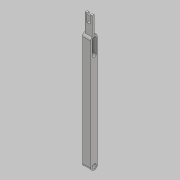
# Autodesk Inventor part: 支架4-15
Saved by Autodesk Inventor 2018 (Build 220112000, 112)
## iProperties
Created: 2021-03-05
Part Number: 支架4-15
Material: 一般
Document SubType Name: Modeling
Designer: 王鼎鈞
Density: 1 g/cm^3
Appearance: 預設
Mass: 2.43299 g
Surface Area: 19.7834 cm^2
Volume: 2.43299 cm^3
Author: 王鼎鈞
Autodesk Inventor part; units mm, degrees
ref_plane "YZ Plane" through (0, 0, 0) normal (1, 0, 0) x (0, 1, 0)
ref_plane "XZ Plane" through (0, 0, 0) normal (0, 1, 0) x (-1, 0, 0)
ref_plane "XY Plane" through (0, 0, 0) normal (0, 0, 1) x (1, 0, 0)
sketch "草圖1" plane through (0, 0, 0) normal (1, 0, 0) x (0, 1, 0)
  line L0 (0, 0) -> (5, 0)
  line L1 (5, 0) -> (5, -85)
  line L2 (5, -85) -> (0, -85)
  line L3 (0, -85) -> (0, 0)
  dimension "d0" = 5
  dimension "d1" = 85
  constraints: 8 end point, 2 parallel, 1 horizontal, 1 perpendicular
  measures "d0" distance of L1.end L2.end
  measures "d1" distance of L0.end L1.end
extrude "擠出1" add sketch "草圖1" along normal blind 6
fillet "圓角1" radius 2.5 2 edges at (3, 5, 0) (3, 0, 0)
hole "孔1" at (6, 2.5, -2.5) direction (-1, 0, 0) diameter 3 end through all
fillet "圓角2" radius 2.5 2 edges at (3, 5, -85) (3, 0, -85)
hole "孔2" at (6, 2.5, -82.5) direction (-1, 0, 0) diameter 3 end through all
sketch "草圖2" plane through (6, 0, 0) normal (1, 0, 0) x (0, 0, -1)
  line L0 (0, -1) -> (0, 6) projected
  line L1 (0, -1) -> (0, 6) projected
  line L2 (120, 0) -> (-20, 0) projected
  circle A0 centre (82.5, 2.5) radius 1.5 projected
  circle A1 centre (2.5, 2.5) radius 1.5 projected
  arc A2 (82.5, 0) -> (82.5, 5) centre (82.5, 2.5) ccw projected
  line L3 (82.5, 5) -> (2.5, 5) projected
  arc A3 (2.5, 5) -> (2.5, 0) centre (2.5, 2.5) ccw projected
  line L4 (2.5, 0) -> (82.5, 0) projected
  circle A4 centre (98.5, 2.5) radius 1.5
  circle A5 centre (82.5, 2.5) radius 1.5 projected
  line L5 (84.5, 4) -> (98.5, 4)
  line L6 (98.5, 4) -> (98.5, 1)
  line L7 (98.5, 1) -> (84.5, 1)
  point P0 (0, 0)
  dimension "d24" = 3
  dimension "d25" = 16
  constraints: 6 end point, 2 point on circle, 1 horizontal, 1 parallel, 1 perpendicular, 1 vertical alignment, 2 other
  measures "d25" distance of A0.centre point (98.5, 2.5)
extrude "擠出2" add sketch "草圖2" against normal blind 5 contours A2 L5 A4 L7 | L6 A4 | A4 L6
ref_plane "工作平面1" through (3, 0, 0) normal (1, 0, 0) x (0, 0, -1)
sketch "草圖3" plane through (3, 0, 0) normal (1, 0, 0) x (0, 0, -1)
  arc A0 (98.5, 1) -> (98.5, 4) centre (98.5, 2.5) ccw projected
  line L0 (98.5, 1) -> (102.8586, 1)
  line L1 (102.8586, 1) -> (102.8586, 5.3685)
  line L2 (102.8586, 5.3685) -> (98.5, 5.3685)
  line L3 (98.5, 5.3685) -> (98.5, 1)
  point P0 (0, 0)
  constraints: 8 end point, 2 parallel, 1 perpendicular
extrude "擠出3" cut sketch "草圖3" along normal mid plane 6
sketch "草圖4" plane through (3, 0, 0) normal (1, 0, 0) x (0, 0, -1)
  line L0 (98.5, 4) -> (98.5, 1) projected
  arc A0 (98.5, 0) -> (98.5, 5) centre (98.5, 2.5) ccw
  line L1 (98.5, 5) -> (98.5, 0)
  point P0 (0, 0)
  dimension "d30" = 5
  constraints: 4 end point, 2 point on circle, 1 centre point, 1 midpoint, 1 vertical
  measures "d30" diameter of A0
revolve "迴轉1" add sketch "草圖4" angle 360 about axis through (3, 5, -98.5) along (0, -1, 0)
ref_plane "工作平面3" through (-79.3581, 2.5, -42.5) normal (0, 0, 1) x (1, 0, 0)
ref_plane "工作平面2" through (-79.3581, 2.5, -2.5) normal (0, 0, 1) x (1, 0, 0)
mirror "鏡射1" about plane through (-79.3581, 2.5, -42.5) normal (0, 0, 1) of "迴轉1", "擠出2", "擠出3"
sketch "草圖5" plane through (0, 0, 0) normal (-1, 0, 0) x (0, 0, 1)
  circle A0 centre (-82.5, 2.5) radius 1.5 projected
  arc A1 (-82.5, 5) -> (-82.5, 0) centre (-82.5, 2.5) ccw projected
  line L0 (-82.5, 0) -> (-2.5, 0) projected
  arc A2 (-2.5, 0) -> (-2.5, 5) centre (-2.5, 2.5) ccw projected
  line L1 (-2.5, 5) -> (-82.5, 5) projected
  circle A3 centre (-2.5, 2.5) radius 1.5 projected
  line L2 (-82.5, 0) -> (-111.7443, 0)
  line L3 (-111.7443, 0) -> (-111.7443, 9.7981)
  line L4 (-111.7443, 9.7981) -> (-82.5, 9.7981)
  line L5 (-82.5, 9.7981) -> (-82.5, 5)
  point P0 (0, 0)
  constraints: 8 end point, 2 parallel, 1 horizontal, 1 perpendicular, 1 point on circle
extrude "擠出4" cut sketch "草圖5" against normal blind 68 contours A1 L2 L3 L4 L5
sketch "草圖6" plane through (6, 4, 13.5) normal (0, 1, 0) x (1, 0, 0)
  line L0 (-5, 14) -> (-5, 0) projected
  line L1 (0, 14) -> (0, 0) projected
  line L2 (-5, 3.7503) -> (0, 3.7503)
  line L3 (0, 3.7503) -> (0, 5.4836)
  line L4 (0, 5.4836) -> (-5, 5.4836)
  line L5 (-5, 5.4836) -> (-5, 3.7503)
  line L6 (-6, 13.5) -> (3.0826, 13.5)
  line L7 (3.0826, 13.5) -> (3.0826, -5.8508)
  line L8 (3.0826, -5.8508) -> (-6, -5.8508)
  line L9 (-6, -5.8508) -> (-6, 13.5)
  dimension "d36" = 1.7333
  constraints: 16 end point, 4 parallel, 2 horizontal, 2 perpendicular, 2 point on line
  measures "d36" distance between parallel lines of L2 L4
extrude "擠出5" cut sketch "草圖6" along normal mid plane 34.75 contours L0 L2 L1 L6 L7 L8 L9 | L0 L6 L1 L4
sketch "草圖7" plane through (1, 4, 9.7497) normal (0, 1, 0) x (1, 0, 0)
  line L0 (6.9259, 3.5729) -> (-0.7883, 3.5729)
  line L1 (-0.7883, 3.5729) -> (-0.7883, -1.5637)
  line L2 (-0.7883, -1.5637) -> (6.9259, -1.5637)
  line L3 (6.9259, -1.5637) -> (6.9259, 3.5729)
  point P0 (-1, 9.7497)
  constraints: 8 end point, 2 parallel, 1 horizontal, 1 perpendicular
extrude "擠出6" cut sketch "草圖7" against normal blind 68.5
sketch "草圖8" plane through (1, 4, 0) normal (0, 0, 1) x (1, 0, 0)
  line L0 (0, -1.5) -> (0, -3) projected
  line L1 (5, 0) -> (5, -3) projected
  line L2 (0, -3) -> (5, -3)
  line L3 (5, -3) -> (5, -1.5)
  line L4 (5, -1.5) -> (0, -1.5)
  line L5 (0, -1.5) -> (0, -3)
  point P0 (-1, -4)
  constraints: 8 end point, 2 parallel, 1 horizontal, 1 midpoint, 1 perpendicular
extrude "擠出7" add sketch "草圖8" along normal blind 13
ref_plane "工作平面5" through (3.5, 0, 0) normal (1, 0, 0) x (0, 0, -1)
sketch "草圖10" plane through (3.5, 0, 0) normal (1, 0, 0) x (0, 0, -1)
  line L0 (-13, 2.5) -> (-13, 1) projected
  arc A0 (-13, 4.5) -> (-13, 0.5) centre (-13, 2.5) ccw
  line L1 (-13, 4.5) -> (-13, 0.5)
  point P0 (0, 0)
  dimension "d45" = 4
  constraints: 2 end point, 2 point on circle, 1 centre point, 1 vertical
  measures "d45" diameter of A0
revolve "迴轉3" add sketch "草圖10" angle 360 about axis through (3.5, 4.5, 13) along (0, -1, 0)
sketch "草圖11" plane through (6, 0, 0) normal (1, 0, 0) x (0, 0, -1)
  circle A0 centre (2.5, 2.5) radius 1.5 projected
  circle A1 centre (82.5, 2.5) radius 1.5 projected
  line L0 (0, 4) -> (0, 2.5) projected
  line L1 (0, 2.5) -> (-13, 2.5) projected
  line L2 (-13, 1) -> (-13, 2.5) projected
  line L3 (0.5, 1) -> (-13, 1) projected
  arc A2 (0.5, 1) -> (2.5, 0) centre (2.5, 2.5) ccw projected
  line L4 (2.5, 0) -> (82.5, 0) projected
  arc A3 (82.5, 0) -> (82.5, 5) centre (82.5, 2.5) ccw projected
  line L5 (82.5, 5) -> (2.5, 5) projected
  arc A4 (2.5, 5) -> (0.5, 4) centre (2.5, 2.5) ccw projected
  line L6 (0, 4) -> (0.5, 4) projected
  circle A5 centre (12.5, 2.5) radius 1.5
  circle A6 centre (2.5, 2.5) radius 1.5 projected
  line L7 (12.5, 1) -> (2.5, 1)
  line L8 (2.5, 1) -> (2.5, 4)
  line L9 (2.5, 4) -> (12.5, 4)
  line L10 (12.5, 4) -> (12.5, 1)
  point P0 (0, 0)
  dimension "d47" = 3
  dimension "d48" = 10
  constraints: 8 end point, 2 parallel, 2 vertical alignment, 1 horizontal, 1 perpendicular, 3 other
  measures "d48" distance of A0.centre point (12.5, 2.5)
extrude "擠出8" cut sketch "草圖11" against normal blind 10 contours A0 L8 | A0 L9 A5 L7 | L10 A5 | A5 L10 picked at (2.7169, 2.9505)
delete faces "刪除面1" heal yes whole lump no faces at (1.6636, 2.5, 13.7922)
sketch "草圖12" plane through (1, 2.5, 13) normal (0, 1, 0) x (1, 0, 0)
  line L0 (5, 0) -> (0, 0) projected
  line L1 (5, 13) -> (5, 0) projected
  line L2 (0, 13) -> (5, 13) projected
  line L3 (0, 13) -> (0, 0) projected
  line L4 (5, 0) -> (0, 0) projected
  line L5 (2.5, 0) -> (2.5, -1.5569)
  line L6 (1.3, 0) -> (3.7, 0)
  line L7 (3.7, 0) -> (3.7, 1.5)
  line L8 (3.7, 1.5) -> (1.3, 1.5)
  line L9 (1.3, 1.5) -> (1.3, 0)
  line L10 (6.3003, 1.5) -> (-1.3715, 1.5)
  line L11 (-1.3715, 1.5) -> (-1.3715, -1.1286)
  line L12 (-1.3715, -1.1286) -> (6.3003, -1.1286)
  line L13 (6.3003, -1.1286) -> (6.3003, 1.5)
  point P0 (-1, 13)
  dimension "d51" = 1.2
  dimension "d52" = 1.5
  constraints: 18 end point, 4 parallel, 2 horizontal, 2 perpendicular, 1 midpoint, 1 point on line, 1 vertical, 1 other
  measures "d51" distance between parallel lines of L5 L7
  measures "d52" distance of L8.end L6.start
extrude "擠出9" cut sketch "草圖12" against normal blind 10 contours L0 L9 L8 L7
sketch "草圖13" plane through (2.3, 2.5, 13) normal (1, 0, 0) x (0, 0, -1)
  line L0 (1.5, -1.5) -> (0, -1.5) projected
  line L1 (1.5, 0) -> (1.5, -1.5) projected
  line L2 (0, 0) -> (1.5, 0) projected
  line L3 (0, -1.5) -> (0, 0) projected
  circle A0 centre (1.5, -0.75) radius 0.25
  point P0 (13, -2.5)
  dimension "d55" = 0.5
  dimension "d56" = 0.75
  dimension "d57" = 1.5
  constraints: 1 centre point
  measures "d55" diameter of A0
  measures "d56" distance from line of L2 A0.centre
  measures "d57" distance from line of L3 A0.centre
extrude "擠出10" add sketch "草圖13" along normal blind 10 contours A0 L1 | L1 A0
delete faces "刪除面2" heal yes whole lump no faces at (8.1, 1.7901, 11.2532)
sketch "草圖14" plane through (1, 2.5, 13) normal (0, 1, 0) x (1, 0, 0)
  line L0 (3.7, 1.5) -> (1.3, 1.5) projected
  line L1 (1.3, 1.5) -> (3.7, 1.5)
  line L2 (3.7, 1.5) -> (3.7, 6)
  line L3 (3.7, 6) -> (1.3, 6)
  line L4 (1.3, 6) -> (1.3, 1.5)
  line L5 (5, 0) -> (3.7, 0) projected
  point P0 (-1, 13)
  dimension "d60" = 6
  constraints: 8 end point, 2 parallel, 1 horizontal, 1 perpendicular
  measures "d60" distance between parallel lines of L5 L3
extrude "擠出11" cut sketch "草圖14" against normal blind 27.5
ref_plane "工作平面4" through (3, 0, -85) normal (-1, 0, 0) x (0, 0, 1)
